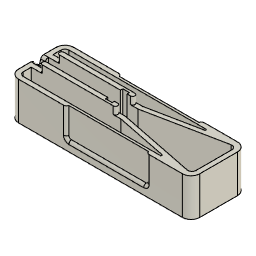
Finale Box oben (Autodesk Fusion 360 design; units mm, degrees)
Autodesk Fusion 360 part; units mm, degrees
note: some values were not read from the file. Set by a fixed rule: which sketch regions a step uses.
sketch "Skizze1" plane through (0, 0, 0) normal (0, 0, 1) x (1, 0, 0)
  line L0 (0, 0) -> (115, 0)
  line L1 (115, 0) -> (115, 35)
  line L2 (115, 35) -> (0, 35)
  line L3 (0, 35) -> (0, 0)
  line L4 (115, 0) -> (115, 35)
  dimension "d1" = 115
  dimension "d2" = 35
  constraint coincident L0.start L3.end
  constraint horizontal L0
  constraint perpendicular L0 L1
  constraint perpendicular L1 L2
  constraint perpendicular L2 L3
  measures "d1" distance of L0.start L0.end
  measures "d2" distance of L0.end L1.end
extrude "Extrusion1" add sketch "Skizze1" along normal blind 8 makes body 1
shell "Schale1" thickness 3 removed faces 1 at (38.3333, 23.3333, 8) on bodies 1
sketch "Skizze2" plane through (0, 0, 3) normal (0, 0, 1) x (-1, 0, 0)
  line L0 (-3, -32) -> (-3, -3)
  line L1 (-3, -3) -> (-112, -3)
  line L2 (-112, -3) -> (-112, -32)
  line L3 (-112, -32) -> (-3, -32)
  line L4 (-67.2609, -10.6) -> (-57, -10.6)
  line L5 (-57, -10.6) -> (-3, -10.6)
  line L6 (-67.2609, -24.4) -> (-3, -24.4)
  line L7 (-62.2103, -13.5) -> (-67.2609, -13.5)
  line L8 (-53.2232, -10.6) -> (-53.2232, -13.5)
  line L9 (-53.2232, -13.5) -> (-3, -13.5)
  line L10 (-53.2232, -13.5) -> (-62.2103, -13.5)
  line L11 (-61, -21.5) -> (-3, -21.5)
  line L12 (-59.8748, -24.4) -> (-59.8748, -32)
  line L13 (-59.8748, -10.6) -> (-59.8748, -3)
  line L14 (-59.8748, -10.6) -> (-59.8748, -24.4)
  line L15 (-59.8748, -13.5) -> (-112, -3)
  line L16 (-59.8748, -10.6) -> (-97.6035, -3)
  line L17 (-59.8748, -21.5) -> (-112, -32)
  line L18 (-59.8748, -24.4) -> (-97.6035, -32)
  line L19 (-97.6035, -3) -> (-112, -3)
  line L20 (-97.6035, -32) -> (-112, -32)
  dimension "d6" = 29
  dimension "d116" = 2.9
  dimension "d118" = 7.6
  dimension "d120" = 7.6
  dimension "d168" = 2.8429
  dimension "d169" = 2.8429
  dimension "d170" = 8
  constraint coincident L0 L5.end
  constraint perpendicular L0 L5
  constraint coincident L0 L6.end
  constraint perpendicular L0 L6
  constraint coincident L5 L8.start
  constraint perpendicular L7 L8
  constraint coincident L0 L9.end
  constraint perpendicular L0 L9
  constraint perpendicular L8 L10
  constraint coincident L0 L11.end
  constraint perpendicular L0 L11
  constraint coincident L6 L12.start
  constraint coincident L3 L12.end
  constraint perpendicular L6 L12
  constraint coincident L4 L13.start
  constraint coincident L1 L13.end
  constraint perpendicular L1 L13
  constraint perpendicular L6 L14
  constraint coincident L14 L15.start
  constraint coincident L10 L15.start
  constraint coincident L1.end L2.start
  constraint coincident L1 L16.end
  constraint parallel L15 L16
  constraint coincident L11 L17.start
  constraint coincident L14 L17.start
  constraint coincident L2.end L3.start
  constraint parallel L17 L18
  constraint perpendicular L2 L20
  measures "d6" distance of L1 L3
  measures "d116" distance of L4.start L7.end
  measures "d118" distance of L1 L5
  measures "d120" distance of L3 L6
  measures "d168" distance of L17 L18
  measures "d169" distance of L15 L16
  measures "d170" distance of L9 L11
extrude "Extrusion2" add sketch "Skizze2" along normal blind 5 contours L0 L6 L11 L14 | L3 L14 L17 L18 L20 | L0 L5 L8 L9 | L4 L5 L8 L10 L14 | L1 L14 L15 L16 L19 bodies 1
extrude "Extrusion3" add 2 faces at (70.8678, 1, 8) (70.8678, 1, 8) along direction (0, 0, 1) blind 1 on bodies 1 bodies 1
sketch "Skizze3" plane through (3, 0, 0) normal (1, 0, 0) x (0, 1, 0)
  line L0 (13.5, 3) -> (21.5, 3)
  line L1 (21.5, 9) -> (13.5, 9)
  line L2 (13.5, 9) -> (21.5, 9)
  line L3 (20, 5.5) -> (15, 5.5)
  line L4 (13.5, 3) -> (21.5, 3)
  line L5 (24.4, 9) -> (24.4, 3)
  line L6 (32, 3) -> (32, 9)
  line L7 (3, 9) -> (3, 3)
  line L8 (32, 9) -> (24.4, 9)
  line L9 (10.6, 3) -> (10.6, 9)
  line L10 (3, 3) -> (10.6, 3)
  line L11 (21.5, 3) -> (21.5, 9)
  line L12 (13.5, 9) -> (13.5, 3)
  line L13 (10.6, 9) -> (3, 9)
  line L14 (24.4, 3) -> (32, 3)
  constraint coincident L1.end L2.start
  constraint coincident L1.start L2.end
  constraint coincident L0.start L4.start
  constraint coincident L0.end L4.end
sketch "Skizze4" plane through (0, 0, 3) normal (0, 0, 1) x (-1, 0, 0)
  line L0 (-37, -15) -> (-37, -16)
  line L1 (-37, -16) -> (-31, -16)
  line L2 (-31, -16) -> (-30, -15)
  line L3 (-37, -20) -> (-37, -19)
  line L4 (-37, -19) -> (-31, -19)
  line L5 (-31, -19) -> (-30, -20)
  line L6 (-112, -3) -> (-112, -32)
  line L7 (-3, -21.5) -> (-3, -13.5)
  line L8 (-37, -15) -> (-37, -14.5)
  line L9 (-30, -15) -> (-30, -14.5)
  line L10 (-30, -20) -> (-30, -20.5)
  line L11 (-37, -20) -> (-37, -20.5)
  line L12 (-112, -32) -> (-59.8748, -21.5)
  line L13 (-59.8748, -21.5) -> (-3, -21.5)
  line L14 (-3, -13.5) -> (-59.8748, -13.5)
  line L15 (-59.8748, -13.5) -> (-112, -3)
  constraint perpendicular L0 L1
  constraint perpendicular L3 L4
sketch "Skizze5" plane through (0, 0, 3) normal (0, 0, 1) x (-1, 0, 0)
  line L0 (-54, -20.4) -> (-54, -19.4)
  line L1 (-54, -19.4) -> (-52, -19.4)
  line L2 (-52, -19.4) -> (-51.5, -20.4)
  line L3 (-54, -15) -> (-54, -16)
  line L4 (-54, -16) -> (-52, -16)
  line L5 (-52, -16) -> (-51.5, -15)
  line L6 (-3, -21.5) -> (-3, -13.5)
  line L7 (-112, -3) -> (-112, -32)
  line L8 (-54, -20.4) -> (-54, -20.5)
  line L9 (-51.5, -20.4) -> (-51.5, -20.5)
  line L10 (-54, -15) -> (-54, -14.9)
  line L11 (-51.5, -15) -> (-51.5, -14.9)
  line L12 (-112, -32) -> (-59.8748, -21.5)
  line L13 (-59.8748, -21.5) -> (-3, -21.5)
  line L14 (-3, -13.5) -> (-59.8748, -13.5)
  line L15 (-59.8748, -13.5) -> (-112, -3)
  constraint perpendicular L0 L1
  constraint perpendicular L3 L4
sketch "Skizze6" plane through (0, 0, 3) normal (0, 0, 1) x (-1, 0, 0)
  line L0 (-59.8748, -10.6) -> (-3, -10.6)
  line L1 (-3, -10.6) -> (-3, -3)
  line L2 (-3, -3) -> (-97.6035, -3)
  line L3 (-3, -10.6) -> (-3, -3)
  line L4 (-97.6035, -3) -> (-59.8748, -10.6)
  line L5 (-97.6035, -3) -> (-59.8748, -10.6)
  constraint coincident L0.end L1.start
  constraint coincident L1.end L2.start
  constraint coincident L2.end L4.start
  constraint coincident L0.start L4.end
sketch "Skizze7" plane through (0, 0, 3) normal (0, 0, 1) x (-1, 0, 0)
  line L0 (-97.6035, -32) -> (-3, -32)
  line L1 (-3, -32) -> (-3, -24.4)
  line L2 (-3, -32) -> (-3, -24.4)
  line L3 (-63, -23) -> (-97.6035, -32)
  line L4 (-3, -24.4) -> (-59.8748, -24.4)
  line L5 (-59.8748, -24.4) -> (-97.6035, -32)
  constraint coincident L0.end L1.start
  constraint coincident L1.end L2.end
  constraint coincident L0.start L3.end
sketch "Skizze8" plane through (0, 0, 9) normal (0, 0, 1) x (-1, 0, 0)
  line L0 (-97.6035, -3) -> (-3, -3)
  line L1 (-3, -13.5) -> (-3, -21.5)
  line L2 (-3, -10.6) -> (-59.8748, -10.6)
  line L3 (-59.8748, -24.4) -> (-3, -24.4)
  line L4 (-3, -32) -> (-97.6035, -32)
  line L5 (0, 0) -> (-115, 0)
  line L6 (-115, 0) -> (-115, -35)
  line L7 (-115, -35) -> (0, -35)
  line L8 (0, -35) -> (0, 0)
  line L9 (-3, -21.5) -> (0, -12)
  line L10 (0, -35) -> (0, -23)
  line L11 (-97.6035, -3) -> (-111.0826, -0.2848)
  line L12 (-97.6035, -32) -> (-113.3045, -35.7715)
  line L13 (-115, -34.7718) -> (-115, 0)
  line L14 (-115, 0) -> (-110, 0)
  line L15 (-110, 0) -> (-97.6035, -3)
  line L16 (-97.6035, -3) -> (-59.8748, -10.6)
  line L17 (-115, -34.7718) -> (-115, -35)
  line L18 (-115, -35) -> (-110, -35)
  line L19 (-110, -35) -> (-97.6035, -32)
  line L20 (-59.8748, -24.4) -> (0, -35)
  line L21 (-59.8748, -10.6) -> (-59.8748, -24.4)
  line L22 (0, -11.8431) -> (0, 0)
  line L23 (-112, -32) -> (-112, -3)
  line L24 (-3, -24.4) -> (-3, -32)
  line L25 (-112, -3) -> (-59.8748, -13.5)
  line L26 (-59.8748, -13.5) -> (-3, -13.5)
  line L27 (-3, -21.5) -> (-59.8748, -21.5)
  line L28 (-59.8748, -21.5) -> (-112, -32)
  line L29 (-97.6035, -32) -> (-59.8748, -24.4)
  line L30 (-3, -3) -> (-3, -10.6)
  line L31 (-59.8748, -10.6) -> (-97.6035, -3)
  dimension "d150" = 3
  dimension "d151" = 3
  constraint coincident L1.end L9.start
  constraint coincident L7.end L8.start
  constraint coincident L0.start L11.start
  constraint coincident L4.end L12.start
  constraint perpendicular L13 L14
  constraint coincident L2.end L16.end
  constraint parallel L13 L17
  constraint perpendicular L17 L18
  constraint coincident L3.start L20.start
  constraint coincident L5.start L8.end
  measures "d150" distance of L4.end L18
  measures "d151" distance of L14 L23.end
extrude "Extrusion11" add sketch "Skizze1" against normal blind 5 separate body makes body 2
fillet "Abrundung11" radius 5.5 4 edges at (115, 0, -2.5) (0, 0, -2.5) (115, 35, -2.5) (0, 35, -2.5) on bodies 2
sketch "Skizze10" plane through (0, 0, 0) normal (0, 0, 1) x (-1, 0, 0)
  arc A0 (-5.5, -35) -> (0, -29.5) centre (-5.5, -29.5) ccw
  line L0 (0, -29.5) -> (0, -5.5)
  arc A1 (0, -5.5) -> (-5.5, 0) centre (-5.5, -5.5) ccw
  line L1 (-5.5, 0) -> (-109.5, 0)
  arc A2 (-109.5, 0) -> (-115, -5.5) centre (-109.5, -5.5) ccw
  line L2 (-115, -5.5) -> (-115, -29.5)
  arc A3 (-115, -29.5) -> (-109.5, -35) centre (-109.5, -29.5) ccw
  line L3 (-109.5, -35) -> (-5.5, -35)
  line L4 (-47, -3) -> (-47, -3.2)
  line L5 (-47, -3.2) -> (-87, -3.2)
  line L6 (-47, -3.2) -> (-10, -3.2)
  line L7 (-10, -3.2) -> (-10, -5.7)
  line L8 (-87, -3.2) -> (-76.0656, -5.7)
  line L9 (-76.0656, -5.7) -> (-10, -5.7)
  line L10 (-10, -32) -> (-10, -31.8)
  line L11 (-10, -31.8) -> (-10, -29.3)
  line L12 (-10, -29.3) -> (-76.0656, -29.3)
  line L13 (-10, -31.8) -> (-90, -31.8)
  line L14 (-87, -31.8) -> (-76.0656, -29.3)
  dimension "d63" = 0.2
  dimension "d64" = 2.5
  dimension "d65" = 0.2
  dimension "d66" = 2.5
  constraint vertical L4
  constraint perpendicular L4 L5
  constraint perpendicular L4 L6
  constraint perpendicular L5 L7
  constraint perpendicular L7 L9
  constraint perpendicular L9 L10
  constraint perpendicular L9 L11
  constraint perpendicular L7 L12
  constraint perpendicular L11 L13
  constraint coincident L13 L14.start
  measures "d63" distance of L4.start L4.end
  measures "d64" distance of L6.end L7.end
  measures "d65" distance of L10.start L10.end
  measures "d66" distance of L10.end L11.end
extrude "Extrusion12" add sketch "Skizze10" along normal blind 5 contours L5 L6 L7 L8 L9 | L11 L12 L13 L14 bodies 2
fillet "Abrundung12" radius 2 1 edges at (10, 29.3, 2.5) on bodies 2
fillet "Abrundung13" radius 2 1 edges at (10, 5.7, 2.5) on bodies 2
fillet "Abrundung14" radius 5 1 edges at (76.0656, 5.7, 2.5) on bodies 2
fillet "Abrundung15" radius 5 1 edges at (76.0656, 29.3, 2.5) on bodies 2
sketch "Skizze11" plane through (0, 0, 3) normal (0, 0, 1) x (-1, 0, 0)
  line L0 (-112, -3) -> (-112, -32)
  line L1 (-62.9948, -20.0432) -> (-62.9948, -14.9568)
  line L2 (-62.9948, -14.9568) -> (-112, -2.9555)
  line L3 (-112, -2.9555) -> (-112, -32)
  line L4 (-112, -32) -> (-62.9948, -20.0432)
  line L5 (-3, -21.5) -> (-3, -13.5)
  line L6 (-112, -32) -> (-59.8748, -21.5)
  line L7 (-59.8748, -21.5) -> (-3, -21.5)
  line L8 (-3, -13.5) -> (-59.8748, -13.5)
  line L9 (-59.8748, -13.5) -> (-112, -3)
  constraint parallel L0 L3
ref_plane "Arbeitsebene1" through (57.5, 17.5, 4) normal (0, 1, 0) x (-1, 0, 0)
sketch "Skizze12" plane through (0, 35, 0) normal (0, 1, 0) x (-1, 0, 0)
  line L0 (-5.5, -5) -> (-5.5, 0)
  line L1 (-5.5, 0) -> (-109.5, 0)
  line L2 (-109.5, 0) -> (-109.5, -5)
  line L3 (-109.5, -5) -> (-5.5, -5)
  line L4 (-36, 0) -> (-36, -1)
  line L5 (-36, -1) -> (-36, -1.5)
  arc A0 (-37.5, -3) -> (-36, -1.5) centre (-37.5, -1.5) ccw
  line L6 (-37.5, -3) -> (-85, -3)
  line L7 (-86.5, -1.5) -> (-86.5, 0)
  arc A1 (-86.5, -1.5) -> (-85, -3) centre (-85, -1.5) ccw
  constraint coincident L1 L4.start
  constraint perpendicular L1 L4
  constraint parallel L4 L5
  constraint tangent L5 A0
  constraint tangent A0 L6
  constraint perpendicular L5 L6
  constraint coincident L1 L7.end
  constraint perpendicular L1 L7
  constraint tangent L6 A1
extrude "Extrusion16" cut sketch "Skizze12" against normal blind 1.5 contours L1 L4 L5 A0 L6 L7 A1 bodies 2
fillet "Abrundung18" radius 2 5 edges at (36, 35, -0.75) (36.4393, 35, -2.5607) (61.25, 35, -3) (86.0607, 35, -2.5607) (86.5, 35, -0.75) on bodies 2
sketch "Skizze13" plane through (0, 35, 0) normal (0, 1, 0) x (-1, 0, 0)
  line L0 (0, 9) -> (-115, 9)
  line L1 (-115, 0) -> (0, 0)
  line L2 (-36, 0) -> (-36, 1.5)
  arc A0 (-36, 1.5) -> (-37.5, 3) centre (-37.5, 1.5) ccw
  line L3 (-83.5, 3) -> (-37.5, 3)
  line L4 (-34, 0) -> (-34, 1.5)
  arc A1 (-34, 1.5) -> (-35.5, 3) centre (-35.5, 1.5) ccw
  line L5 (-35.5, 3) -> (-38.5, 3)
  line L6 (-86.5, 0) -> (-86.5, 1.5)
  arc A2 (-85, 3) -> (-86.5, 1.5) centre (-85, 1.5) ccw
  line L7 (-85, 3) -> (-83.5, 3)
  line L8 (0, 0) -> (0, 9)
  line L9 (-115, 9) -> (-115, 0)
  constraint coincident L1 L2.start
  constraint perpendicular L1 L2
  constraint tangent L2 A0
  constraint coincident L1 L4.start
  constraint perpendicular L1 L4
  constraint tangent L4 A1
  constraint coincident L3 L5.end
  constraint tangent A1 L5
  constraint perpendicular L4 L5
  constraint coincident L1 L6.start
  constraint perpendicular L1 L6
  constraint tangent L6 A2
sketch "Skizze9" plane through (0, 0, 9) normal (0, 0, 1) x (-1, 0, 0)
  line L0 (-97.6035, -3) -> (-3, -3)
  line L1 (-3, -13.5) -> (-3, -21.5)
  line L2 (-3, -10.6) -> (-59.8748, -10.6)
  line L3 (-59.8748, -24.4) -> (-3, -24.4)
  line L4 (-3, -32) -> (-97.6035, -32)
  line L5 (0, 0) -> (-115, 0)
  line L6 (-115, 0) -> (-115, -35)
  line L7 (-115, -35) -> (0, -35)
  line L8 (0, -35) -> (0, 0)
  line L9 (-112, -32) -> (-112, -3)
  line L10 (-97.6035, -3) -> (-97.6035, -32)
  line L11 (-97.6035, -32) -> (-59.8748, -24.4)
  line L12 (-59.8748, -10.6) -> (-97.6035, -3)
  line L13 (-59.8748, -10.6) -> (-59.8748, -24.4)
  line L14 (-115, 0) -> (-115, -35)
  line L15 (-115, -35) -> (-110, -35)
  line L16 (-110, -35) -> (-97.6035, -32)
  line L17 (-115, 0) -> (-110, 0)
  line L18 (-110, 0) -> (-97.6035, -3)
  line L19 (-3, -24.4) -> (-3, -32)
  line L20 (-112, -3) -> (-59.8748, -13.5)
  line L21 (-59.8748, -13.5) -> (-3, -13.5)
  line L22 (-3, -21.5) -> (-59.8748, -21.5)
  line L23 (-59.8748, -21.5) -> (-112, -32)
  line L24 (-97.6035, -32) -> (-59.8748, -24.4)
  line L25 (-3, -3) -> (-3, -10.6)
  line L26 (-59.8748, -10.6) -> (-97.6035, -3)
  constraint coincident L0.start L10.start
  constraint coincident L4.end L10.end
  constraint coincident L3.start L11.end
  constraint coincident L2.end L12.start
  constraint parallel L6 L14
  constraint perpendicular L14 L15
  constraint perpendicular L14 L17
sketch "Skizze14" plane through (0, 0, 0) normal (0, -1, 0) x (1, 0, 0)
  line L0 (0, 0) -> (115, 0)
  line L1 (115, 9) -> (0, 9)
  line L2 (36, 0) -> (36, 1.5)
  arc A0 (37.5, 3) -> (36, 1.5) centre (37.5, 1.5) ccw
  line L3 (37.5, 3) -> (85, 3)
  line L4 (86.5, 0) -> (86.5, 1.5)
  arc A1 (86.5, 1.5) -> (85, 3) centre (85, 1.5) ccw
  line L5 (115, 0) -> (115, 9)
  line L6 (0, 9) -> (0, 0)
  constraint coincident L0 L2.start
  constraint perpendicular L0 L2
  constraint tangent L2 A0
  constraint tangent A0 L3
  constraint perpendicular L2 L3
  constraint coincident L0 L4.start
  constraint perpendicular L0 L4
  constraint tangent L4 A1
  constraint tangent L3 A1
sketch "Skizze15" plane through (0, 0, 0) normal (0, -1, 0) x (1, 0, 0)
  line L0 (5.5, 0) -> (5.5, -5)
  line L1 (5.5, -5) -> (109.5, -5)
  line L2 (109.5, -5) -> (109.5, 0)
  line L3 (109.5, 0) -> (5.5, 0)
  line L4 (36, 0) -> (36, -1.5)
  arc A0 (36, -1.5) -> (37.5, -3) centre (37.5, -1.5) ccw
  line L5 (37.5, -3) -> (86.5, -3)
  line L6 (86.5, 0) -> (86.5, -1.5)
  arc A1 (85, -3) -> (86.5, -1.5) centre (85, -1.5) ccw
  constraint coincident L3 L4.start
  constraint perpendicular L3 L4
  constraint tangent L4 A0
  constraint tangent A0 L5
  constraint perpendicular L4 L5
  constraint coincident L3 L6.start
  constraint perpendicular L3 L6
  constraint coincident L5 A1.start
  constraint tangent L6 A1
extrude "Extrusion19" cut sketch "Skizze15" against normal blind 1.5 contours L3 L4 A0 L5 L6 A1 bodies 2
fillet "Abrundung21" radius 2 5 edges at (86.5, 0, -0.75) (86.0607, 0, -2.5607) (61.25, 0, -3) (36.4393, 0, -2.5607) (36, 0, -0.75) on bodies 2
sketch "Skizze16" plane through (0, 0, 0) normal (0, -1, 0) x (1, 0, 0)
  line L0 (115, 9) -> (0, 9)
  line L1 (0, 0) -> (115, 0)
  line L2 (36, 9) -> (36, 7.5)
  arc A0 (36, 7.5) -> (37.5, 6) centre (37.5, 7.5) ccw
  line L3 (37.5, 6) -> (85, 6)
  arc A1 (85, 6) -> (86.5, 7.5) centre (85, 7.5) ccw
  line L4 (86.5, 7.5) -> (86.5, 9)
  line L5 (115, 0) -> (115, 9)
  line L6 (0, 9) -> (0, 0)
  constraint coincident L0 L2.start
  constraint perpendicular L0 L2
  constraint tangent L2 A0
  constraint tangent A0 L3
  constraint tangent L3 A1
  constraint tangent A1 L4
extrude "Extrusion20" cut sketch "Skizze16" against normal blind 1.5 contours L0 L2 A0 L3 A1 L4 bodies 1
sketch "Skizze17" plane through (0, 35, 0) normal (0, 1, 0) x (-1, 0, 0)
  line L0 (0, 9) -> (-115, 9)
  line L1 (-115, 0) -> (0, 0)
  line L2 (-36, 9) -> (-36, 7.5)
  arc A0 (-37.5, 6) -> (-36, 7.5) centre (-37.5, 7.5) ccw
  line L3 (-37.5, 6) -> (-85, 6)
  arc A1 (-86.5, 7.5) -> (-85, 6) centre (-85, 7.5) ccw
  line L4 (-86.5, 7.5) -> (-86.5, 9)
  line L5 (0, 0) -> (0, 9)
  line L6 (-115, 9) -> (-115, 0)
  constraint coincident L0 L2.start
  constraint perpendicular L0 L2
  constraint tangent L2 A0
  constraint tangent A0 L3
  constraint perpendicular L2 L3
  constraint tangent L3 A1
  constraint coincident L0 L4.end
  constraint tangent A1 L4
  constraint perpendicular L0 L4
extrude "Extrusion21" cut sketch "Skizze17" against normal blind 1.5 contours L0 L2 A0 L3 A1 L4 bodies 1
fillet "Abrundung23" radius 2 5 edges at (36, 35, 8.25) (36.4393, 35, 6.4393) (61.25, 35, 6) (86.0607, 35, 6.4393) (86.5, 35, 8.25) on bodies 1
fillet "Abrundung24" radius 2 5 edges at (86.5, 0, 8.25) (86.0607, 0, 6.4393) (61.25, 0, 6) (36.4393, 0, 6.4393) (36, 0, 8.25) on bodies 1
sketch "Skizze18" plane through (0, 0, 0) normal (-1, 0, 0) x (0, -1, 0)
  line L0 (0, 9) -> (-35, 9)
  line L1 (-35, 0) -> (0, 0)
  line L2 (-17.5, 0) -> (-17.5, 9)
  line L3 (-17.5, 9) -> (-20.1, 9)
  line L4 (-17.5, 9) -> (-14.9, 9)
  line L5 (-20.1, 9) -> (-20.1, 0)
  line L6 (-14.9, 9) -> (-14.9, 0)
  line L7 (-17.5, 9) -> (-17.5, 7.7767)
  line L8 (-20.1, 7.9804) -> (-14.9, 7.9804)
  line L9 (-17.5, 4.5) -> (-20.1, 4.5)
  line L10 (-17.5, 4.5) -> (-14.9, 4.5)
  line L11 (0, 0) -> (0, 9)
  line L12 (-35, 9) -> (-35, 0)
  dimension "d131" = 2.6
  dimension "d132" = 2.6
  dimension "d134" = 3.4804
  constraint midpoint L1 L2.start
  constraint midpoint L0 L2.end
  constraint perpendicular L2 L3
  constraint perpendicular L2 L4
  constraint coincident L1 L5.end
  constraint perpendicular L1 L5
  constraint coincident L1 L6.end
  constraint perpendicular L1 L6
  constraint coincident L2 L7.end
  constraint coincident L5 L8.start
  constraint coincident L6 L8.end
  constraint perpendicular L6 L8
  constraint midpoint L2 L9.start
  constraint midpoint L5 L9.end
  constraint midpoint L6 L10.end
  measures "d131" distance of L2.end L3.end
  measures "d132" distance of L2.end L4.end
  measures "d134" distance of L8 L9
sketch "Skizze19" plane through (3, 0, 0) normal (1, 0, 0) x (0, 1, 0)
  line L0 (24.4, 3) -> (32, 3)
  line L1 (32, 9) -> (24.4, 9)
  line L2 (24.4, 3) -> (24.4, 12.0395)
  line L3 (32, 12.0395) -> (32, 3)
  line L4 (24.4, 12.0395) -> (32, 12.0395)
  line L5 (24.4, 3) -> (32, 3)
  line L6 (21.5, 3) -> (21.5, 9)
  line L7 (13.5, 9) -> (13.5, 3)
  line L8 (10.6, 3) -> (10.6, 9)
  line L9 (10.6, 9) -> (3, 9)
  line L10 (3, 9) -> (3, 3)
  line L11 (3, 3) -> (10.6, 3)
  line L12 (24.4, 9) -> (24.4, 3)
  line L13 (32, 3) -> (32, 9)
  line L14 (21.5, 9) -> (13.5, 9)
  line L15 (13.5, 3) -> (21.5, 3)
  constraint coincident L0.start L2.start
  constraint perpendicular L0 L2
  constraint coincident L0.end L3.end
  constraint perpendicular L0 L3
  constraint perpendicular L3 L4
extrude "Extrusion22" add 1 faces at (1, 18.8333, 9) along direction (0, 0, 1) blind 15 on bodies 1 bodies 1
fillet "Abrundung32" radius 1 1 edges at (87, 31.8, 2.5) on bodies 2
fillet "Abrundung33" radius 1 1 edges at (87, 3.2, 2.5) on bodies 2
fillet "Abrundung34" radius 1 1 edges at (10, 3.2, 2.5) on bodies 2
fillet "Abrundung35" radius 1 1 edges at (10, 31.8, 2.5) on bodies 2
fillet "Abrundung38" radius 2.5 4 edges at (3, 32, 13.5) (112, 3, 13.5) (3, 3, 13.5) (112, 32, 13.5) on bodies 1
fillet "Abrundung39" radius 5.5 4 edges at (0, 0, 12) (0, 35, 12) (115, 35, 12) (115, 0, 12) on bodies 1
fillet "Abrundung40" radius 0.5 2 edges at (97.6035, 3, 13.5) (97.6035, 32, 13.5) on bodies 1
sketch "Skizze20" plane through (0, 0, 3) normal (0, 0, 1) x (-1, 0, 0)
  line L0 (-59.8748, -21.5) -> (-3, -21.5)
  line L1 (-3, -13.5) -> (-59.8748, -13.5)
  line L2 (-75, -24.5468) -> (-75, -10.4532)
  line L3 (-57.4759, -24.6) -> (-10.0118, -24.6)
  line L4 (-10, -21.5) -> (-10, -21.3)
  line L5 (-10, -21.3) -> (-10, -24.6)
  line L6 (-10, -24.6) -> (-10.0118, -24.6)
  line L7 (-10, -21.3) -> (-55, -21.3)
  line L8 (-55, -21.3) -> (-55, -24.6)
  line L9 (-49, -13.5) -> (-49, -13.7)
  line L10 (-47.5, -10.6) -> (-47.5, -10.4)
  line L11 (-55, -10.4) -> (-55, -13.5)
  line L12 (-55, -13.5) -> (-55, -13.7)
  line L13 (-55, -13.7) -> (-49, -13.7)
  line L14 (-55, -10.4) -> (-47.5, -10.4)
  line L15 (-49, -13.7) -> (-10, -13.7)
  line L16 (-10, -13.7) -> (-10, -10.4)
  line L17 (-10, -10.4) -> (-47.5, -10.4)
  arc A0 (-10, -13.7) -> (-10, -10.4) centre (-10, -12.05) ccw
  arc A1 (-55, -10.4) -> (-55, -13.7) centre (-55, -12.05) ccw
  arc A2 (-55, -21.3) -> (-55, -24.6) centre (-55, -22.95) ccw
  arc A3 (-10, -24.6) -> (-10, -21.3) centre (-10, -22.95) ccw
  arc A4 (-112, -28.9462) -> (-109.0063, -31.397) centre (-109.5, -28.9462) ccw
  line L18 (-109.0063, -31.397) -> (-59.8748, -21.5)
  line L19 (-3, -21.5) -> (-3, -13.5)
  line L20 (-59.8748, -13.5) -> (-109.0063, -3.603)
  arc A5 (-109.0063, -3.603) -> (-112, -6.0538) centre (-109.5, -6.0538) ccw
  line L21 (-112, -6.0538) -> (-112, -28.9462)
  dimension "d188" = 0.2
  dimension "d189" = 45
  dimension "d190" = 0.2
  constraint vertical L2
  constraint perpendicular L1 L4
  constraint perpendicular L3 L5
  constraint perpendicular L5 L6
  constraint perpendicular L5 L7
  constraint coincident L3 L8.end
  constraint perpendicular L3 L8
  constraint vertical L9
  constraint vertical L10
  constraint perpendicular L7 L11
  constraint perpendicular L7 L12
  constraint perpendicular L9 L13
  constraint perpendicular L10 L14
  constraint perpendicular L4 L15
  constraint perpendicular L15 L16
  constraint perpendicular L10 L17
  constraint tangent L15 A0
  constraint tangent L13 A1
  constraint tangent L7 A2
  constraint tangent L7 A3
  measures "d188" distance of L4.start L4.end
  measures "d189" distance of L4.end L7.end
  measures "d190" distance of L9.start L9.end
extrude "Extrusion27" cut sketch "Skizze20" against normal blind 11 contours L2 A4 L18 L20 A5 L21 bodies 1
sketch "Skizze21" plane through (0, 24.4, 0) normal (0, 1, 0) x (-1, 0, 0)
  line L0 (-3, 3) -> (-3, 24)
  line L1 (-3, 24) -> (-59.8748, 24)
  line L2 (-59.8748, 24) -> (-59.8748, 3)
  line L3 (-25, 0) -> (-25, 3)
  line L4 (-25, 3) -> (-3, 3)
  line L5 (-59.8748, 3) -> (-3, 3)
  constraint coincident L0 L4.end
  constraint perpendicular L0 L4
sketch "Skizze22" plane through (0, 0, 0) normal (0, 0, 1) x (-1, 0, 0)
  line L0 (-11.134, -31.8) -> (-78.1396, -31.8)
  arc A0 (-78.3625, -29.8252) -> (-78.1396, -31.8) centre (-78.1396, -30.8) ccw
  line L1 (-78.3625, -29.8252) -> (-76.6157, -29.4258)
  arc A1 (-75.5013, -29.3) -> (-76.6157, -29.4258) centre (-75.5013, -34.3) ccw
  line L2 (-75.5013, -29.3) -> (-12, -29.3)
  arc A2 (-10.2679, -30.3) -> (-12, -29.3) centre (-12, -31.3) ccw
  arc A3 (-11.134, -31.8) -> (-10.2679, -30.3) centre (-11.134, -30.8) ccw
  arc A4 (-12, -5.7) -> (-10.2679, -4.7) centre (-12, -3.7) ccw
  line L3 (-12, -5.7) -> (-75.5013, -5.7)
  arc A5 (-76.6157, -5.5742) -> (-75.5013, -5.7) centre (-75.5013, -0.7) ccw
  line L4 (-76.6157, -5.5742) -> (-78.3625, -5.1748)
  arc A6 (-78.1396, -3.2) -> (-78.3625, -5.1748) centre (-78.1396, -4.2) ccw
  line L5 (-78.1396, -3.2) -> (-11.134, -3.2)
  arc A7 (-10.2679, -4.7) -> (-11.134, -3.2) centre (-11.134, -4.2) ccw
  arc A8 (-86.5, -1.5) -> (-88.4365, 0) centre (-88.4365, -2) ccw
  line L6 (-88.4365, 0) -> (-109.5, 0)
  arc A9 (-109.5, 0) -> (-115, -5.5) centre (-109.5, -5.5) ccw
  line L7 (-115, -5.5) -> (-115, -29.5)
  arc A10 (-115, -29.5) -> (-109.5, -35) centre (-109.5, -29.5) ccw
  line L8 (-109.5, -35) -> (-88.4365, -35)
  arc A11 (-88.4365, -35) -> (-86.5, -33.5) centre (-88.4365, -33) ccw
  line L9 (-86.5, -33.5) -> (-36, -33.5)
  arc A12 (-36, -33.5) -> (-34.0635, -35) centre (-34.0635, -33) ccw
  line L10 (-34.0635, -35) -> (-5.5, -35)
  arc A13 (-5.5, -35) -> (0, -29.5) centre (-5.5, -29.5) ccw
  line L11 (0, -29.5) -> (0, -5.5)
  arc A14 (0, -5.5) -> (-5.5, 0) centre (-5.5, -5.5) ccw
  line L12 (-5.5, 0) -> (-34.0635, 0)
  arc A15 (-34.0635, 0) -> (-36, -1.5) centre (-34.0635, -2) ccw
  line L13 (-36, -1.5) -> (-86.5, -1.5)
  line L14 (-49, -13.5) -> (-49, -13.7)
  line L15 (-49, -13.7) -> (-55, -13.7)
  line L16 (-47.5, -10.6) -> (-47.5, -10.4)
  line L17 (-47.5, -10.4) -> (-55, -10.4)
  arc A16 (-55, -10.4) -> (-55, -13.7) centre (-55, -12.05) ccw
  line L18 (-47.5, -10.4) -> (-10, -10.4)
  arc A17 (-10, -13.7) -> (-10, -10.4) centre (-10, -12.05) ccw
  line L19 (-10, -13.7) -> (-49, -13.7)
  line L20 (-55, -21.3) -> (-51.6, -21.3)
  line L21 (-51.6, -21.3) -> (-55, -21.3)
  arc A18 (-55, -21.3) -> (-55, -24.6) centre (-55, -22.95) ccw
  line L22 (-55, -24.6) -> (-10, -24.6)
  arc A19 (-10, -24.6) -> (-10, -21.3) centre (-10, -22.95) ccw
  line L23 (-10, -21.3) -> (-51.6, -21.3)
  dimension "d191" = 0.2
  constraint perpendicular L3 L14
  constraint perpendicular L14 L15
  constraint vertical L16
  constraint perpendicular L16 L17
  constraint tangent L17 A16
  constraint perpendicular L16 L18
  constraint tangent L18 A17
  constraint tangent A17 L19
  constraint perpendicular L16 L20
  constraint tangent L20 A18
  constraint tangent A18 L22
  constraint parallel L21 L22
  constraint tangent L22 A19
  constraint tangent A19 L23
  measures "d191" distance of L14.start L14.end
extrude "Extrusion28" cut sketch "Skizze22" against normal blind 5 contours L15 L17 A16 L18 A17 L19 | L20 L21 A18 L22 A19 L23 bodies 2
sketch "Skizze23" plane through (0, 0, 24) normal (0, 0, 1) x (-1, 0, 0)
  line L0 (-59.8748, -21.5) -> (-109.0063, -31.397)
  arc A0 (-112, -28.9462) -> (-109.0063, -31.397) centre (-109.5, -28.9462) ccw
  line L1 (-112, -28.9462) -> (-112, -6.0538)
  arc A1 (-109.0063, -3.603) -> (-112, -6.0538) centre (-109.5, -6.0538) ccw
  line L2 (-109.0063, -3.603) -> (-59.8748, -13.5)
  line L3 (-92.6881, -31.0098) -> (-59.8748, -24.4)
  line L4 (-59.8748, -24.4) -> (-3, -24.4)
  line L5 (-3, -24.4) -> (-3, -29.5)
  arc A2 (-5.5, -32) -> (-3, -29.5) centre (-5.5, -29.5) ccw
  line L6 (-5.5, -32) -> (-92.5894, -32)
  arc A3 (-92.6881, -31.0098) -> (-92.5894, -32) centre (-92.5894, -31.5) ccw
  line L7 (-3, -10.6) -> (-59.8748, -10.6)
  line L8 (-59.8748, -10.6) -> (-92.6881, -3.9902)
  arc A4 (-92.5894, -3) -> (-92.6881, -3.9902) centre (-92.5894, -3.5) ccw
  line L9 (-92.5894, -3) -> (-5.5, -3)
  arc A5 (-3, -5.5) -> (-5.5, -3) centre (-5.5, -5.5) ccw
  line L10 (-3, -13.5) -> (-3, -21.5)
  arc A6 (-109.5, 0) -> (-115, -5.5) centre (-109.5, -5.5) ccw
  line L11 (-115, -5.5) -> (-115, -29.5)
  arc A7 (-115, -29.5) -> (-109.5, -35) centre (-109.5, -29.5) ccw
  line L12 (-109.5, -35) -> (-88.4365, -35)
  arc A8 (-88.4365, -35) -> (-86.5, -33.5) centre (-88.4365, -33) ccw
  line L13 (-86.5, -33.5) -> (-36, -33.5)
  arc A9 (-36, -33.5) -> (-34.0635, -35) centre (-34.0635, -33) ccw
  line L14 (-34.0635, -35) -> (-5.5, -35)
  arc A10 (-5.5, -35) -> (0, -29.5) centre (-5.5, -29.5) ccw
  line L15 (0, -29.5) -> (0, -5.5)
  arc A11 (0, -5.5) -> (-5.5, 0) centre (-5.5, -5.5) ccw
  line L16 (-5.5, 0) -> (-34.0635, 0)
  arc A12 (-34.0635, 0) -> (-36, -1.5) centre (-34.0635, -2) ccw
  line L17 (-36, -1.5) -> (-86.5, -1.5)
  arc A13 (-86.5, -1.5) -> (-88.4365, 0) centre (-88.4365, -2) ccw
  line L18 (-88.4365, 0) -> (-109.5, 0)
  line L19 (-10, -23) -> (-10, -24.4)
  line L20 (-10, -21.5) -> (-55, -21.5)
  line L21 (-55, -24.4) -> (-10, -24.4)
  line L22 (-10, -24.4) -> (-10, -21.5)
  line L23 (-55, -24.4) -> (-55, -21.5)
  line L24 (-10, -13.5) -> (-10, -10.6)
  line L25 (-55, -10.6) -> (-55, -13.5)
  line L26 (-10, -13.5) -> (-55, -13.5)
  line L27 (-55, -10.6) -> (-10, -10.6)
  arc A14 (-10, -13.5) -> (-10, -10.6) centre (-10, -12.05) ccw
  arc A15 (-10, -24.4) -> (-10, -21.5) centre (-10, -22.95) ccw
  arc A16 (-55, -21.5) -> (-55, -24.4) centre (-55, -22.95) ccw
  arc A17 (-55, -10.6) -> (-55, -13.5) centre (-55, -12.05) ccw
  line L28 (-59.8748, -13.5) -> (-3, -13.5)
  line L29 (-3, -21.5) -> (-59.8748, -21.5)
  line L30 (-3, -5.5) -> (-3, -10.6)
  constraint coincident L4 L19.end
  constraint perpendicular L4 L19
  constraint perpendicular L19 L20
  constraint coincident L4 L21.start
  constraint coincident L7 L24.end
  constraint perpendicular L7 L24
  constraint coincident L7 L25.start
  constraint tangent L27 A14
  constraint tangent L20 A15
  constraint tangent L21 A15
  constraint tangent L20 A16
  constraint tangent L26 A17
  constraint tangent L27 A17
extrude "Extrusion29" add sketch "Skizze23" along normal blind 4.8 contours L4 L19 L20 L21 L22 L23 L29 | L23 A16 | L19 L22 A15 | L7 L24 L25 L26 L27 L28 | L24 A14 | L25 A17 bodies 1
sketch "Skizze24" plane through (0, 0, 3) normal (0, 0, 1) x (-1, 0, 0)
  line L0 (-54.9894, -21.5) -> (-50.7894, -21.5)
  line L1 (-50.7894, -13.5) -> (-54.9894, -13.5)
  line L2 (-50.7894, -13.5) -> (-50.7894, -14)
  line L3 (-50.7894, -21.5) -> (-50.7894, -22.5)
  line L4 (-54.9894, -22.5) -> (-54.9894, -21.5)
  line L5 (-54.9894, -12) -> (-54.9894, -13.5)
  line L6 (-52.8894, -21.5) -> (-52.8894, -13.5)
  line L7 (-52.8894, -13.5) -> (-48.6894, -13.5)
  line L8 (-48.6894, -21.5) -> (-52.8894, -21.5)
  line L9 (-48.6894, -21.5) -> (-48.6894, -13.5)
  line L10 (-48.6894, -13.5) -> (-48.6894, -12)
  line L11 (-48.6894, -12) -> (-52.8894, -12)
  line L12 (-52.8894, -12) -> (-52.8894, -21.5)
  line L13 (-48.6894, -21.5) -> (-48.6894, -23)
  line L14 (-48.6894, -23) -> (-52.8894, -23)
  line L15 (-52.8894, -23) -> (-52.8894, -21.5)
  line L16 (-3, -21.5) -> (-3, -13.5)
  line L17 (-75, -10.4532) -> (-75, -24.5468)
  line L18 (-75, -24.5468) -> (-59.8748, -21.5)
  line L19 (-59.8748, -21.5) -> (-3, -21.5)
  line L20 (-3, -13.5) -> (-59.8748, -13.5)
  line L21 (-59.8748, -13.5) -> (-75, -10.4532)
  dimension "d196" = 4.2
  dimension "d199" = 4.2
  constraint perpendicular L1 L2
  constraint perpendicular L0 L3
  constraint midpoint L0 L6.start
  constraint midpoint L1 L6.end
  constraint perpendicular L1 L6
  constraint perpendicular L6 L7
  constraint perpendicular L6 L8
  constraint perpendicular L7 L9
  constraint perpendicular L7 L10
  constraint perpendicular L6 L11
  constraint perpendicular L8 L12
  constraint perpendicular L8 L13
  constraint perpendicular L13 L14
  constraint perpendicular L8 L15
  measures "d196" distance of L0.start L0.end
  measures "d199" distance of L6.end L7.end
extrude "Extrusion30" cut sketch "Skizze24" along normal blind 29 contours L0 L1 L6 L12 L17 L18 L19 L20 L21 | L0 L1 L6 L7 L8 L9 L12 L19 L20 | L0 L8 L13 L14 L15 L19 bodies 1
extrude "Extrusion31" cut sketch "Skizze24" along normal blind 31 and the other way blind 5 contours L0 L1 L6 L7 L8 L9 L12 L19 L20 | L0 L8 L13 L14 L15 L19 | L1 L7 L10 L11 L12 L20 bodies 1
sketch "Skizze25" plane through (0, 0, 0) normal (0, 0, 1) x (-1, 0, 0)
  arc A0 (-55, -21.3) -> (-55, -24.6) centre (-55, -22.95) ccw
  line L0 (-55, -21.3) -> (-10, -21.3)
  arc A1 (-10, -24.6) -> (-10, -21.3) centre (-10, -22.95) ccw
  line L1 (-10, -24.6) -> (-55, -24.6)
  arc A2 (-55, -10.4) -> (-55, -13.7) centre (-55, -12.05) ccw
  line L2 (-55, -10.4) -> (-10, -10.4)
  arc A3 (-10, -13.7) -> (-10, -10.4) centre (-10, -12.05) ccw
  line L3 (-10, -13.7) -> (-55, -13.7)
  line L4 (-11.134, -31.8) -> (-78.1396, -31.8)
  arc A4 (-78.3625, -29.8252) -> (-78.1396, -31.8) centre (-78.1396, -30.8) ccw
  line L5 (-78.3625, -29.8252) -> (-76.6157, -29.4258)
  arc A5 (-75.5013, -29.3) -> (-76.6157, -29.4258) centre (-75.5013, -34.3) ccw
  line L6 (-75.5013, -29.3) -> (-12, -29.3)
  arc A6 (-10.2679, -30.3) -> (-12, -29.3) centre (-12, -31.3) ccw
  arc A7 (-11.134, -31.8) -> (-10.2679, -30.3) centre (-11.134, -30.8) ccw
  arc A8 (-12, -5.7) -> (-10.2679, -4.7) centre (-12, -3.7) ccw
  line L7 (-12, -5.7) -> (-75.5013, -5.7)
  arc A9 (-76.6157, -5.5742) -> (-75.5013, -5.7) centre (-75.5013, -0.7) ccw
  line L8 (-76.6157, -5.5742) -> (-78.3625, -5.1748)
  arc A10 (-78.1396, -3.2) -> (-78.3625, -5.1748) centre (-78.1396, -4.2) ccw
  line L9 (-78.1396, -3.2) -> (-11.134, -3.2)
  arc A11 (-10.2679, -4.7) -> (-11.134, -3.2) centre (-11.134, -4.2) ccw
  arc A12 (-86.5, -1.5) -> (-88.4365, 0) centre (-88.4365, -2) ccw
  line L10 (-88.4365, 0) -> (-109.5, 0)
  arc A13 (-109.5, 0) -> (-115, -5.5) centre (-109.5, -5.5) ccw
  line L11 (-115, -5.5) -> (-115, -29.5)
  arc A14 (-115, -29.5) -> (-109.5, -35) centre (-109.5, -29.5) ccw
  line L12 (-109.5, -35) -> (-88.4365, -35)
  arc A15 (-88.4365, -35) -> (-86.5, -33.5) centre (-88.4365, -33) ccw
  line L13 (-86.5, -33.5) -> (-36, -33.5)
  arc A16 (-36, -33.5) -> (-34.0635, -35) centre (-34.0635, -33) ccw
  line L14 (-34.0635, -35) -> (-5.5, -35)
  arc A17 (-5.5, -35) -> (0, -29.5) centre (-5.5, -29.5) ccw
  line L15 (0, -29.5) -> (0, -5.5)
  arc A18 (0, -5.5) -> (-5.5, 0) centre (-5.5, -5.5) ccw
  line L16 (-5.5, 0) -> (-34.0635, 0)
  arc A19 (-34.0635, 0) -> (-36, -1.5) centre (-34.0635, -2) ccw
  line L17 (-36, -1.5) -> (-86.5, -1.5)
  line L18 (-48.6895, -21.3) -> (-48.6895, -13.7)
  line L19 (-48.6895, -13.7) -> (-52.8895, -13.7)
  line L20 (-52.8895, -13.7) -> (-52.8895, -21.3)
  line L21 (-48.6895, -21.3) -> (-52.8895, -21.3)
  dimension "d202" = 4.2
  constraint coincident L0 L18.start
  constraint coincident L3 L18.end
  constraint perpendicular L3 L18
  constraint perpendicular L18 L19
  constraint coincident L0 L20.end
  constraint perpendicular L0 L20
  measures "d202" distance of L18.end L19.end
extrude "Extrusion32" cut sketch "Skizze25" against normal blind 3 contours L0 L3 L18 L19 L20 L21 bodies 2
sketch "Skizze28" plane through (0, 0, 0) normal (0, 0, 1) x (-1, 0, 0)
  arc A0 (-86.5, -1.5) -> (-88.4365, 0) centre (-88.4365, -2) ccw
  line L0 (-88.4365, 0) -> (-109.5, 0)
  arc A1 (-109.5, 0) -> (-115, -5.5) centre (-109.5, -5.5) ccw
  line L1 (-115, -5.5) -> (-115, -29.5)
  arc A2 (-115, -29.5) -> (-109.5, -35) centre (-109.5, -29.5) ccw
  line L2 (-109.5, -35) -> (-88.4365, -35)
  arc A3 (-88.4365, -35) -> (-86.5, -33.5) centre (-88.4365, -33) ccw
  line L3 (-86.5, -33.5) -> (-36, -33.5)
  arc A4 (-36, -33.5) -> (-34.0635, -35) centre (-34.0635, -33) ccw
  line L4 (-34.0635, -35) -> (-5.5, -35)
  arc A5 (-5.5, -35) -> (0, -29.5) centre (-5.5, -29.5) ccw
  line L5 (0, -29.5) -> (0, -5.5)
  arc A6 (0, -5.5) -> (-5.5, 0) centre (-5.5, -5.5) ccw
  line L6 (-5.5, 0) -> (-34.0635, 0)
  arc A7 (-34.0635, 0) -> (-36, -1.5) centre (-34.0635, -2) ccw
  line L7 (-36, -1.5) -> (-86.5, -1.5)
  arc A8 (-12, -5.7) -> (-10.2679, -4.7) centre (-12, -3.7) ccw
  line L8 (-12, -5.7) -> (-75.5013, -5.7)
  arc A9 (-76.6157, -5.5742) -> (-75.5013, -5.7) centre (-75.5013, -0.7) ccw
  line L9 (-76.6157, -5.5742) -> (-78.3625, -5.1748)
  arc A10 (-78.1396, -3.2) -> (-78.3625, -5.1748) centre (-78.1396, -4.2) ccw
  line L10 (-78.1396, -3.2) -> (-11.134, -3.2)
  arc A11 (-10.2679, -4.7) -> (-11.134, -3.2) centre (-11.134, -4.2) ccw
  line L11 (-11.134, -31.8) -> (-78.1396, -31.8)
  arc A12 (-78.3625, -29.8252) -> (-78.1396, -31.8) centre (-78.1396, -30.8) ccw
  line L12 (-78.3625, -29.8252) -> (-76.6157, -29.4258)
  arc A13 (-75.5013, -29.3) -> (-76.6157, -29.4258) centre (-75.5013, -34.3) ccw
  line L13 (-75.5013, -29.3) -> (-12, -29.3)
  arc A14 (-10.2679, -30.3) -> (-12, -29.3) centre (-12, -31.3) ccw
  arc A15 (-11.134, -31.8) -> (-10.2679, -30.3) centre (-11.134, -30.8) ccw
  line L14 (-52.8895, -21.3) -> (-52.8895, -13.7)
  line L15 (-52.8895, -13.7) -> (-55, -13.7)
  arc A16 (-55, -10.4) -> (-55, -13.7) centre (-55, -12.05) ccw
  line L16 (-55, -10.4) -> (-10, -10.4)
  arc A17 (-10, -13.7) -> (-10, -10.4) centre (-10, -12.05) ccw
  line L17 (-10, -13.7) -> (-48.6895, -13.7)
  line L18 (-48.6895, -13.7) -> (-48.6895, -21.3)
  line L19 (-48.6895, -21.3) -> (-10, -21.3)
  arc A18 (-10, -24.6) -> (-10, -21.3) centre (-10, -22.95) ccw
  line L20 (-10, -24.6) -> (-55, -24.6)
  arc A19 (-55, -21.3) -> (-55, -24.6) centre (-55, -22.95) ccw
  line L21 (-55, -21.3) -> (-52.8895, -21.3)
  line L22 (-75, -24.5) -> (-75, -10.5)
  line L23 (-75, -10.5) -> (-112, -3)
  line L24 (-75, -24.5) -> (-112, -32)
  line L25 (-112, -32) -> (-112, -3)
  constraint perpendicular L8 L22
  constraint parallel L1 L25
sketch "Skizze26" plane through (0, 0, 0) normal (-1, 0, 0) x (0, -1, 0)
  line L0 (-29.5, 24) -> (-29.5, 0)
  line L1 (-29.5, 0) -> (-5.5, 0)
  line L2 (-5.5, 0) -> (-5.5, 24)
  line L3 (-5.5, 24) -> (-29.5, 24)
  line L4 (-18.8867, 20) -> (-16.1424, 20)
  line L5 (-16.1424, 20) -> (-15.0033, 24)
  line L6 (-18.8867, 20) -> (-20, 24)
  dimension "d205" = 4
  constraint coincident L3 L5.end
  constraint coincident L3 L6.end
  measures "d205" distance of L3 L4
extrude "Extrusion33" cut sketch "Skizze26" against normal blind 3.5 contours L3 L4 L5 L6 bodies 1
fillet "Abrundung43" radius 2 2 edges at (1.5, 20, 24) (1.5, 15.0033, 24) on bodies 1
fillet "Abrundung44" radius 0.75 2 edges at (1.5, 18.8867, 20) (1.5, 16.1424, 20) on bodies 1
fillet "Abrundung46" radius 5.5 2 edges at (75, 24.5468, 1.5) (75, 10.4532, 1.5) on bodies 1
extrude "Extrusion34" cut sketch "Skizze28" against normal blind 2 contours L22 L23 L24 L25 bodies 2
fillet "Abrundung47" radius 2.5 2 edges at (112, 32, -1) (112, 3, -1) on bodies 2
fillet "Abrundung48" radius 3 2 edges at (75, 10.5, -1) (75, 24.5, -1) on bodies 2
sketch "Skizze29" plane through (0, 0, 0) normal (0, 0, -1) x (1, 0, 0)
  line L0 (52.8894, -23) -> (48.6894, -23)
  line L1 (48.6894, -23) -> (48.6894, -12)
  line L2 (48.6894, -12) -> (52.8894, -12)
  line L3 (52.8894, -12) -> (52.8894, -23)
  arc A0 (109.0063, -31.397) -> (112, -28.9462) centre (109.5, -28.9462) ccw
  line L4 (109.0063, -31.397) -> (79.4139, -25.4359)
  arc A1 (75, -20.0442) -> (79.4139, -25.4359) centre (80.5, -20.0442) ccw
  line L5 (75, -20.0442) -> (75, -14.9558)
  arc A2 (79.4139, -9.5641) -> (75, -14.9558) centre (80.5, -14.9558) ccw
  line L6 (79.4139, -9.5641) -> (109.0063, -3.603)
  arc A3 (112, -6.0538) -> (109.0063, -3.603) centre (109.5, -6.0538) ccw
  line L7 (112, -6.0538) -> (112, -28.9462)
  arc A4 (115, -5.5) -> (109.5, 0) centre (109.5, -5.5) ccw
  line L8 (109.5, 0) -> (5.5, 0)
  arc A5 (5.5, 0) -> (0, -5.5) centre (5.5, -5.5) ccw
  line L9 (0, -5.5) -> (0, -29.5)
  arc A6 (0, -29.5) -> (5.5, -35) centre (5.5, -29.5) ccw
  line L10 (5.5, -35) -> (109.5, -35)
  arc A7 (109.5, -35) -> (115, -29.5) centre (109.5, -29.5) ccw
  line L11 (115, -29.5) -> (115, -5.5)
  line L12 (52.8894, -14.027) -> (55.8894, -14.027)
  line L13 (52.8894, -12) -> (55.8894, -12)
  line L14 (55.8894, -12) -> (55.8894, -14.027)
  line L15 (52.8894, -23) -> (55.8894, -23)
  line L16 (55.8894, -23) -> (55.8894, -20.973)
  line L17 (55.8894, -20.973) -> (52.8894, -20.973)
  line L18 (55.8894, -20.973) -> (55.8894, -14.027)
  line L19 (55.8894, -14.027) -> (52.8894, -12)
  line L20 (55.8894, -20.973) -> (52.8894, -23)
  line L21 (48.6894, -20.973) -> (45.6894, -20.973)
  line L22 (45.6894, -20.973) -> (45.6894, -14.027)
  line L23 (45.6894, -14.027) -> (48.6894, -14.027)
  line L24 (45.6894, -20.973) -> (48.6894, -23)
  line L25 (45.6894, -14.027) -> (48.6894, -12)
  dimension "d231" = 3
  dimension "d232" = 2.027
  dimension "d233" = 3
  constraint coincident L3 L12.start
  constraint perpendicular L3 L12
  constraint coincident L2.end L3.start
  constraint perpendicular L3 L13
  constraint perpendicular L12 L14
  constraint coincident L0.start L3.end
  constraint perpendicular L14 L15
  constraint perpendicular L15 L16
  constraint coincident L3 L17.end
  constraint perpendicular L3 L17
  constraint perpendicular L12 L18
  constraint coincident L1 L21.start
  constraint perpendicular L1 L21
  constraint perpendicular L12 L22
  constraint coincident L1 L23.end
  constraint perpendicular L1 L23
  constraint coincident L0.end L1.start
  constraint coincident L1.end L2.start
  measures "d231" distance of L12.start L12.end
  measures "d232" distance of L15.end L16.end
  measures "d233" distance of L21.start L21.end
extrude "Extrusion35" cut sketch "Skizze29" against normal blind 2 contours L3 L17 L20 | L1 L21 L24 | L3 L12 L17 L18 | L1 L21 L22 L23 | L3 L12 L19 | L1 L23 L25 bodies 1
sketch "Skizze30" plane through (0, 0, 0) normal (0, 0, -1) x (1, 0, 0)
  line L0 (45.6894, -14.027) -> (48.6894, -12)
  line L1 (48.6894, -12) -> (52.8894, -12)
  line L2 (52.8894, -12) -> (55.8894, -14.027)
  line L3 (55.8894, -14.027) -> (55.8894, -20.973)
  line L4 (55.8894, -20.973) -> (52.8894, -23)
  line L5 (52.8894, -23) -> (48.6894, -23)
  line L6 (48.6894, -23) -> (45.6894, -20.973)
  line L7 (45.6894, -20.973) -> (45.6894, -14.027)
  arc A0 (109.0063, -31.397) -> (112, -28.9462) centre (109.5, -28.9462) ccw
  line L8 (109.0063, -31.397) -> (79.4139, -25.4359)
  arc A1 (75, -20.0442) -> (79.4139, -25.4359) centre (80.5, -20.0442) ccw
  line L9 (75, -20.0442) -> (75, -14.9558)
  arc A2 (79.4139, -9.5641) -> (75, -14.9558) centre (80.5, -14.9558) ccw
  line L10 (79.4139, -9.5641) -> (109.0063, -3.603)
  arc A3 (112, -6.0538) -> (109.0063, -3.603) centre (109.5, -6.0538) ccw
  line L11 (112, -6.0538) -> (112, -28.9462)
  arc A4 (115, -5.5) -> (109.5, 0) centre (109.5, -5.5) ccw
  line L12 (109.5, 0) -> (5.5, 0)
  arc A5 (5.5, 0) -> (0, -5.5) centre (5.5, -5.5) ccw
  line L13 (0, -5.5) -> (0, -29.5)
  arc A6 (0, -29.5) -> (5.5, -35) centre (5.5, -29.5) ccw
  line L14 (5.5, -35) -> (109.5, -35)
  arc A7 (109.5, -35) -> (115, -29.5) centre (109.5, -29.5) ccw
  line L15 (115, -29.5) -> (115, -5.5)
  line L16 (48.6894, -12) -> (38, -15)
  line L17 (38, -15) -> (38, -20)
  line L18 (38, -20) -> (48.6894, -23)
  line L19 (52.8894, -23) -> (62, -20)
  line L20 (52.8894, -12) -> (62, -15)
  line L21 (62, -15) -> (62, -20)
  dimension "d246" = 5
  dimension "d247" = 10.6894
  dimension "d248" = 10.6894
  constraint coincident L0.end L1.start
  constraint perpendicular L1 L17
  constraint coincident L5.end L6.start
  constraint coincident L4.end L5.start
  constraint coincident L1.end L2.start
  constraint parallel L3 L21
  measures "d246" distance of L16.end L17.end
  measures "d247" horizontal distance of L0.end L16.end
  measures "d248" horizontal distance of L17.end L5.end
extrude "Extrusion36" cut sketch "Skizze30" against normal blind 2 contours L0 L6 L7 L16 L17 L18 | L0 L1 L2 L3 L4 L5 L6 L7 | L2 L3 L4 L19 L20 L21 bodies 1
fillet "Abrundung54" radius 3.5 2 edges at (38, 20, 1) (38, 15, 1) on bodies 1
fillet "Abrundung55" radius 3.5 2 edges at (62, 15, 1) (62, 20, 1) on bodies 1
chamfer "Fase6" distance 2 angle 45 8 edges at (44.8943, 13.0651, 0) (44.8943, 21.9349, 0) (38.545, 17.5, 0) (56.1929, 13.0878, 0) (61.9017, 17.5, 0) (56.1929, 21.9122, 0) (50.7894, 12, 0) (50.7894, 23, 0) on bodies 1
sketch "Skizze31" plane through (0, 0, 0) normal (0, 0, -1) x (1, 0, 0)
  arc A0 (109.0063, -31.397) -> (112, -28.9462) centre (109.5, -28.9462) ccw
  line L0 (109.0063, -31.397) -> (79.4139, -25.4359)
  arc A1 (75, -20.0442) -> (79.4139, -25.4359) centre (80.5, -20.0442) ccw
  line L1 (75, -20.0442) -> (75, -14.9558)
  arc A2 (79.4139, -9.5641) -> (75, -14.9558) centre (80.5, -14.9558) ccw
  line L2 (79.4139, -9.5641) -> (109.0063, -3.603)
  arc A3 (112, -6.0538) -> (109.0063, -3.603) centre (109.5, -6.0538) ccw
  line L3 (112, -6.0538) -> (112, -28.9462)
  arc A4 (115, -5.5) -> (109.5, 0) centre (109.5, -5.5) ccw
  line L4 (109.5, 0) -> (5.5, 0)
  arc A5 (5.5, 0) -> (0, -5.5) centre (5.5, -5.5) ccw
  line L5 (0, -5.5) -> (0, -29.5)
  arc A6 (0, -29.5) -> (5.5, -35) centre (5.5, -29.5) ccw
  line L6 (5.5, -35) -> (109.5, -35)
  arc A7 (109.5, -35) -> (115, -29.5) centre (109.5, -29.5) ccw
  line L7 (115, -29.5) -> (115, -5.5)
  line L8 (53.2102, -25) -> (48.4141, -25)
  line L9 (48.4141, -25) -> (40.5588, -22.7954)
  arc A8 (40.5588, -12.2046) -> (40.5588, -22.7954) centre (42.045, -17.5) ccw
  line L10 (40.5588, -12.2046) -> (48.4141, -10)
  line L11 (48.4141, -10) -> (53.2102, -10)
  line L12 (53.2102, -10) -> (60.1219, -12.2759)
  arc A9 (60.1219, -22.7241) -> (60.1219, -12.2759) centre (58.4017, -17.5) ccw
  line L13 (60.1219, -22.7241) -> (53.2102, -25)
  line L14 (12, -2) -> (5, -2)
  arc A10 (5, -2) -> (2, -5) centre (5, -5) ccw
  line L15 (2, -5) -> (2, -30)
  arc A11 (2, -30) -> (5, -33) centre (5, -30) ccw
  line L16 (5, -33) -> (16, -33)
  line L17 (16, -33) -> (16, -32)
  line L18 (16, -32) -> (5, -32)
  arc A12 (3, -30) -> (5, -32) centre (5, -30) ccw
  line L19 (3, -30) -> (3, -5)
  arc A13 (5, -3) -> (3, -5) centre (5, -5) ccw
  line L20 (5, -3) -> (12, -3)
  line L21 (12, -3) -> (12, -2)
  line L22 (12, -2) -> (16, -2)
  constraint parallel L4 L14
  constraint tangent L14 A10
  constraint tangent A10 L15
  constraint perpendicular L14 L15
  constraint tangent L15 A11
  constraint tangent A11 L16
  constraint perpendicular L15 L16
  constraint perpendicular L16 L17
  constraint perpendicular L15 L18
  constraint tangent L18 A12
  constraint tangent A12 L19
  constraint perpendicular L16 L19
  constraint tangent L19 A13
  constraint tangent A13 L20
  constraint perpendicular L19 L20
  constraint perpendicular L14 L21
  constraint perpendicular L17 L22
fillet "Abrundung52" [suppressed]
fillet "Abrundung53" [suppressed]
copy_body "Körper->Berechn1" [suppressed] in component "Component"
copy_body "Körper->Berechn2" [suppressed] in component "Component'"
sketch "Skizze27" plane through (0, 0, 0) normal (0, 0, 1) x (-1, 0, 0)
  arc A0 (-86.5, -1.5) -> (-88.4365, 0) centre (-88.4365, -2) ccw
  line L0 (-88.4365, 0) -> (-109.5, 0)
  arc A1 (-109.5, 0) -> (-115, -5.5) centre (-109.5, -5.5) ccw
  line L1 (-115, -5.5) -> (-115, -29.5)
  arc A2 (-115, -29.5) -> (-109.5, -35) centre (-109.5, -29.5) ccw
  line L2 (-109.5, -35) -> (-88.4365, -35)
  arc A3 (-88.4365, -35) -> (-86.5, -33.5) centre (-88.4365, -33) ccw
  line L3 (-86.5, -33.5) -> (-36, -33.5)
  arc A4 (-36, -33.5) -> (-34.0635, -35) centre (-34.0635, -33) ccw
  line L4 (-34.0635, -35) -> (-5.5, -35)
  arc A5 (-5.5, -35) -> (0, -29.5) centre (-5.5, -29.5) ccw
  line L5 (0, -29.5) -> (0, -5.5)
  arc A6 (0, -5.5) -> (-5.5, 0) centre (-5.5, -5.5) ccw
  line L6 (-5.5, 0) -> (-34.0635, 0)
  arc A7 (-34.0635, 0) -> (-36, -1.5) centre (-34.0635, -2) ccw
  line L7 (-36, -1.5) -> (-86.5, -1.5)
  arc A8 (-12, -5.7) -> (-10.2679, -4.7) centre (-12, -3.7) ccw
  line L8 (-12, -5.7) -> (-75.5013, -5.7)
  arc A9 (-76.6157, -5.5742) -> (-75.5013, -5.7) centre (-75.5013, -0.7) ccw
  line L9 (-76.6157, -5.5742) -> (-78.3625, -5.1748)
  arc A10 (-78.1396, -3.2) -> (-78.3625, -5.1748) centre (-78.1396, -4.2) ccw
  line L10 (-78.1396, -3.2) -> (-11.134, -3.2)
  arc A11 (-10.2679, -4.7) -> (-11.134, -3.2) centre (-11.134, -4.2) ccw
  line L11 (-11.134, -31.8) -> (-78.1396, -31.8)
  arc A12 (-78.3625, -29.8252) -> (-78.1396, -31.8) centre (-78.1396, -30.8) ccw
  line L12 (-78.3625, -29.8252) -> (-76.6157, -29.4258)
  arc A13 (-75.5013, -29.3) -> (-76.6157, -29.4258) centre (-75.5013, -34.3) ccw
  line L13 (-75.5013, -29.3) -> (-12, -29.3)
  arc A14 (-10.2679, -30.3) -> (-12, -29.3) centre (-12, -31.3) ccw
  arc A15 (-11.134, -31.8) -> (-10.2679, -30.3) centre (-11.134, -30.8) ccw
  line L14 (-52.8895, -21.3) -> (-52.8895, -13.7)
  line L15 (-52.8895, -13.7) -> (-55, -13.7)
  arc A16 (-55, -10.4) -> (-55, -13.7) centre (-55, -12.05) ccw
  line L16 (-55, -10.4) -> (-10, -10.4)
  arc A17 (-10, -13.7) -> (-10, -10.4) centre (-10, -12.05) ccw
  line L17 (-10, -13.7) -> (-48.6895, -13.7)
  line L18 (-48.6895, -13.7) -> (-48.6895, -21.3)
  line L19 (-48.6895, -21.3) -> (-10, -21.3)
  arc A18 (-10, -24.6) -> (-10, -21.3) centre (-10, -22.95) ccw
  line L20 (-10, -24.6) -> (-55, -24.6)
  arc A19 (-55, -21.3) -> (-55, -24.6) centre (-55, -22.95) ccw
  line L21 (-55, -21.3) -> (-52.8895, -21.3)
extrude "Extrusion13" [suppressed]
extrude "Extrusion14" [suppressed]
extrude "Extrusion10" [suppressed]
fillet "Abrundung10" [suppressed]
hidden bodies 2
